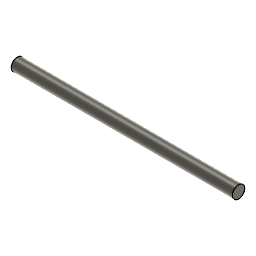
ax (Autodesk Fusion 360 design; units mm, degrees)
part number: 2026-06-02-10-52-54-374
Autodesk Fusion 360 part; units mm, degrees
sketch "Ax" plane through (0, 0, 0) normal (1, 0, 0) x (0, 1, 0)
  circle A0 centre (0, 0) radius 2.25
  dimension "d1" = 4.5
  constraint coincident A0.centre origin
  measures "d1" diameter of A0
extrude "Extrude1" add sketch "Ax" along normal blind 80
named bodies: "Ax"
